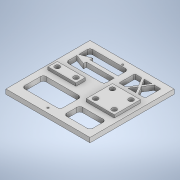
# Autodesk Inventor part: HallSensor_Halterung
Saved by Autodesk Inventor 2022.2 (Build 262287010, 287A)
## iProperties
Created: 2024-01-10
Part Number: HallSensor_Halterung
Material: Generisch
Document SubType Name: Modeling
Designer: ppovolni
Density: 1 g/cm^3
Appearance: Vorgabe
Author: ppovolni
Autodesk Inventor part; units mm, degrees
ref_plane "YZ Plane" through (0, 0, 0) normal (1, 0, 0) x (0, 1, 0)
ref_plane "Arbeitsebene1" through (-21.4485, 99.4, 5.4) normal (-1, 0, 0) x (0, -0.6026, -0.798)
sketch "center1" plane through (-21.4485, 99.4, 5.4) normal (-1, 0, 0) x (0, -0.6026, -0.798)
  line L0 (125.8462, -4.4299) -> (-42.8597, 122.9603)
  line L1 (111.6965, 152.237) -> (-23.2865, -26.5243)
  point P0 (64.2081, 76.0713)
  constraints: 4 end point, 6 other
ref_plane "Arbeitsebene2" through (53.5515, 27.1, 8) normal (0, 0, -1) x (0, 1, 0)
sketch "center2" plane through (53.5515, 27.1, 8) normal (0, 0, -1) x (0, 1, 0)
  line L0 (0, 239.86) -> (0, -220.81)
  point P0 (-27.1, -53.5515)
  constraints: 2 end point, 1 vertical, 2 other
sketch "Hallsensor" plane through (0, 0, 0) normal (0, 1, 0) x (-1, 0, 0)
  line L0 (21.4485, 13) -> (41.4485, 13) construction
  line L1 (41.4485, 13) -> (41.4485, 3) construction
  line L2 (41.4485, 3) -> (21.4485, 3) construction
  line L3 (21.4485, 3) -> (21.4485, 13) construction
  line L4 (21.4485, -97.7) -> (21.4485, 113.7) construction
  line L5 (-293.4115, 8) -> (167.2585, 8) construction
  line L6 (40.4485, 4) -> (42.4485, 4)
  line L7 (42.4485, 4) -> (42.4485, 2)
  line L8 (42.4485, 2) -> (40.4485, 2)
  line L9 (40.4485, 2) -> (40.4485, 4)
  line L10 (40.4485, 4) -> (42.4485, 2) construction
  line L11 (42.4485, 4) -> (40.4485, 2) construction
  line L12 (22.4485, 4) -> (20.4485, 4)
  line L13 (20.4485, 4) -> (20.4485, 2)
  line L14 (20.4485, 2) -> (22.4485, 2)
  line L15 (22.4485, 2) -> (22.4485, 4)
  line L16 (22.4485, 4) -> (20.4485, 2) construction
  line L17 (20.4485, 4) -> (22.4485, 2) construction
  line L18 (22.4485, 14) -> (20.4485, 14)
  line L19 (20.4485, 14) -> (20.4485, 12)
  line L20 (20.4485, 12) -> (22.4485, 12)
  line L21 (22.4485, 12) -> (22.4485, 14)
  line L22 (22.4485, 14) -> (20.4485, 12) construction
  line L23 (20.4485, 14) -> (22.4485, 12) construction
  line L24 (42.4485, 14) -> (40.4485, 14)
  line L25 (40.4485, 14) -> (40.4485, 12)
  line L26 (40.4485, 12) -> (42.4485, 12)
  line L27 (42.4485, 12) -> (42.4485, 14)
  line L28 (42.4485, 14) -> (40.4485, 12) construction
  line L29 (40.4485, 14) -> (42.4485, 12) construction
  line L30 (51.4485, -1) -> (1.4485, -1) construction
  line L31 (1.4485, -1) -> (1.4485, 17) construction
  line L32 (1.4485, 17) -> (51.4485, 17) construction
  line L33 (51.4485, 17) -> (51.4485, -1) construction
  circle A0 centre (51.4485, 8) radius 1.5
  circle A1 centre (1.4485, -1) radius 1.5
  circle A2 centre (1.4485, 17) radius 1.5
  point P0 (0, 0)
  point P1 (21.4485, 3)
  point P2 (21.4485, 3)
  dimension "d70" = 20
  dimension "d71" = 10
  dimension "d72" = 2
  dimension "d73" = 4
  dimension "d74" = 4
  dimension "d75" = 20
  dimension "d76" = 10
  dimension "d77" = 3
  dimension "d78" = 5
  constraints: 64 end point, 12 midpoint, 12 parallel, 6 equal length, 6 horizontal, 6 perpendicular, 3 centre point, 3 coincident, 2 equal radius, 1 collinear, 1 point on line
  measures "d70" distance of L1.end L2.end
  measures "d71" distance of L0.end L1.end
  measures "d72" distance of L7.end L8.end
  measures "d73" distance from line of point (21.448, 3) L30
  measures "d74" distance from line of L32 point (21.448, 13)
  measures "d75" distance from line of point (21.448, 3) L31
  measures "d76" distance between parallel lines of L33 L1
  measures "d77" diameter of A0
  measures "d78" distance between parallel lines of L5 L2
sketch "Groundplane" plane through (0, 0, 0) normal (0, 1, 0) x (-1, 0, 0)
  line L0 (-293.4115, 8) -> (167.2585, 8) construction
  line L1 (21.4485, -97.7) -> (21.4485, 113.7) construction
  arc A0 (22.4485, -32) -> (20.4485, -32) centre (21.4485, -32) ccw construction
  line L2 (22.4485, -32) -> (20.4485, -32) construction
  line L3 (20.4485, -32) -> (20.4485, -37) construction
  line L4 (20.4485, -37) -> (22.4485, -37) construction
  line L5 (22.4485, -37) -> (22.4485, -32) construction
  arc A1 (20.4485, 48) -> (22.4485, 48) centre (21.4485, 48) ccw construction
  line L6 (20.4485, 48) -> (22.4485, 48) construction
  line L7 (22.4485, 48) -> (22.4485, 53) construction
  line L8 (22.4485, 53) -> (20.4485, 53) construction
  line L9 (20.4485, 53) -> (20.4485, 48) construction
  line L10 (61.4485, -37) -> (-28.5515, -37) construction
  line L11 (-28.5515, -37) -> (-28.5515, 53) construction
  line L12 (-28.5515, 53) -> (61.4485, 53) construction
  line L13 (61.4485, 53) -> (61.4485, -37) construction
  dimension "d87" = 5
  dimension "d88" = 2
  dimension "d89" = 2
  dimension "d90" = 5
  dimension "d91" = 90
  dimension "d92" = 45
  dimension "d97" = 50
  dimension "d98" = 90
  constraints: 24 end point, 6 parallel, 5 point on circle, 4 point on line, 3 horizontal, 3 perpendicular, 2 centre point, 2 collinear, 2 midpoint
  measures "d87" distance of L4.end L2.start
  measures "d88" distance of L3.end L4.end
  measures "d89" distance of L7.end L8.end
  measures "d90" distance of L6.end L7.end
  measures "d91" distance of L12.end L10.start
  measures "d92" distance between parallel lines of L0 L10
  measures "d97" distance between parallel lines of L1 L11
  measures "d98" distance of L10.start L10.end
sketch "Montagepunkte" plane through (0, 0, 0) normal (0, 1, 0) x (-1, 0, 0)
  circle A0 centre (51.4485, 8) radius 1.5 construction
  circle A1 centre (1.4485, -1) radius 1.5 construction
  circle A2 centre (1.4485, 17) radius 1.5 construction
  line L0 (1.4485, -1) -> (-18.5515, -1) construction
  line L1 (-18.5515, -1) -> (-18.5515, 17) construction
  line L2 (-18.5515, 17) -> (1.4485, 17) construction
  line L3 (1.4485, 17) -> (1.4485, -1) construction
  line L4 (51.4485, 8) -> (31.4485, 8) construction
  circle A3 centre (31.4485, 8) radius 1.6
  circle A4 centre (51.4485, 8) radius 1.6
  circle A5 centre (1.4485, -1) radius 1.6
  circle A6 centre (1.4485, 17) radius 1.6
  circle A7 centre (-18.5515, 17) radius 1.6
  circle A8 centre (-18.5515, -1) radius 1.6
  arc A9 (22.4485, -32) -> (20.4485, -32) centre (21.4485, -32) ccw construction
  arc A10 (20.4485, 48) -> (22.4485, 48) centre (21.4485, 48) ccw construction
  circle A11 centre (21.4485, -32) radius 1
  circle A12 centre (21.4485, 48) radius 1
  dimension "d93" = 20
  dimension "d94" = 20
  dimension "d95" = 3.2
  dimension "d96" = 2
  constraints: 10 end point, 8 centre point, 8 coincident, 6 equal radius, 2 horizontal, 2 parallel, 1 perpendicular, 1 point on line
  measures "d93" distance of L0.start L0.end
  measures "d94" distance of L4.start L4.end
  measures "d95" diameter of A4
  measures "d96" diameter of A11
sketch "Skizze5" plane through (0, 0, 0) normal (0, 1, 0) x (-1, 0, 0)
  line L0 (-293.4115, 8) -> (167.2585, 8) construction
  circle A0 centre (21.4485, -32) radius 1 projected
  circle A1 centre (21.4485, 48) radius 1 projected
  line L1 (61.4485, -37) -> (-28.5515, -37) projected
  line L2 (61.4485, 53) -> (61.4485, -37) projected
  line L3 (-28.5515, -37) -> (-28.5515, 53) projected
  line L4 (-28.5515, 53) -> (61.4485, 53) projected
extrude "Extrusion2" add sketch "Skizze5" along normal blind 5
sketch "Skizze6" plane through (0, 5, 0) normal (0, 1, 0) x (1, 0, 0)
  line L0 (-56.4485, -3) -> (-26.4485, -3)
  line L1 (-26.4485, -3) -> (-26.4485, -13)
  line L2 (-26.4485, -13) -> (-56.4485, -13)
  line L3 (-56.4485, -13) -> (-56.4485, -3)
  line L4 (-6.4485, 6) -> (23.5515, 6)
  line L5 (23.5515, 6) -> (23.5515, -22)
  line L6 (23.5515, -22) -> (-6.4485, -22)
  line L7 (-6.4485, -22) -> (-6.4485, 6)
  circle A0 centre (-51.4485, -8) radius 1.6 projected
  circle A1 centre (-31.4485, -8) radius 1.6 projected
  circle A2 centre (-1.4485, -17) radius 1.6 projected
  circle A3 centre (18.5515, -17) radius 1.6 projected
  circle A4 centre (18.5515, 1) radius 1.6 projected
  circle A5 centre (-1.4485, 1) radius 1.6 projected
  point P0 (0, 0)
  dimension "d99" = 5
  dimension "d100" = 5
  dimension "d101" = 5
  dimension "d102" = 5
  dimension "d103" = 5
  dimension "d104" = 5
  dimension "d105" = 5
  dimension "d106" = 5
  constraints: 16 end point, 4 parallel, 2 horizontal, 2 perpendicular
  measures "d99" distance from line of A0.centre L0
  measures "d100" distance from line of L2 A0.centre
  measures "d101" distance from line of A1.centre L1
  measures "d102" distance from line of L3 A0.centre
  measures "d103" distance from line of L7 A5.centre
  measures "d104" distance from line of L5 A4.centre
  measures "d105" distance from line of A4.centre L4
  measures "d106" distance from line of L6 A3.centre
extrude "Extrusion3" add sketch "Skizze6" along normal blind 3
chamfer "Fase1" distance 1 distance2 3 2 edges at (-53.0485, 8, 8) (-33.0485, 8, 8) measured on face at (-38.3043, 8, 4.168)
chamfer "Fase2" distance 1 distance2 3 4 edges at (-3.0485, 8, -1) (16.9515, 8, -1) (16.9515, 8, 17) (-3.0485, 8, 17) measured on face at (11.4857, 8, 5.3537)
sketch "Skizze7" plane through (0, 5, 0) normal (0, 1, 0) x (1, 0, 0)
  line L0 (-51.4505, 30) -> (-16.4485, 30)
  line L1 (-13.4485, 27) -> (-13.4485, 7)
  line L2 (-16.4485, 4) -> (-51.4505, 4)
  line L3 (-54.4505, 7) -> (-54.4505, 27)
  line L4 (-51.4505, -20) -> (-16.4485, -20)
  line L5 (-13.4485, -23) -> (-13.4485, -40)
  line L6 (-16.4485, -43) -> (-51.4505, -43)
  line L7 (-54.4505, -40) -> (-54.4505, -23)
  line L8 (-3.4485, -29) -> (18.5497, -29)
  line L9 (21.5497, -32) -> (21.5497, -43)
  line L10 (18.5497, -46) -> (-3.4485, -46)
  line L11 (-6.4485, -43) -> (-6.4485, -32)
  line L12 (28.5497, -53) -> (28.5497, 37)
  line L13 (-61.4505, -53) -> (28.5497, -53)
  line L14 (-61.4505, 37) -> (-61.4505, -53)
  line L15 (-56.4485, -13) -> (-26.4485, -13) projected
  line L16 (-6.4485, 6) -> (-6.4485, -22) projected
  line L17 (-26.4485, -3) -> (-56.4485, -3) projected
  line L18 (28.5497, 37) -> (-61.4505, 37)
  line L19 (-6.4485, -22) -> (23.5515, -22) projected
  line L20 (-5.4485, 30) -> (20.5497, 30)
  line L21 (21.5497, 29) -> (21.5497, 14)
  line L22 (20.5497, 13) -> (-5.4485, 13)
  line L23 (-6.4485, 14) -> (-6.4485, 29)
  line L24 (23.5515, 6) -> (-6.4485, 6) projected
  arc A0 (-51.4505, 30) -> (-54.4505, 27) centre (-51.4505, 27) ccw
  arc A1 (-54.4505, 7) -> (-51.4505, 4) centre (-51.4505, 7) ccw
  arc A2 (-13.4485, 27) -> (-16.4485, 30) centre (-16.4485, 27) ccw
  arc A3 (-16.4485, 4) -> (-13.4485, 7) centre (-16.4485, 7) ccw
  arc A4 (-51.4505, -20) -> (-54.4505, -23) centre (-51.4505, -23) ccw
  arc A5 (-13.4485, -23) -> (-16.4485, -20) centre (-16.4485, -23) ccw
  arc A6 (-16.4485, -43) -> (-13.4485, -40) centre (-16.4485, -40) ccw
  arc A7 (-54.4505, -40) -> (-51.4505, -43) centre (-51.4505, -40) ccw
  arc A8 (-3.4485, -29) -> (-6.4485, -32) centre (-3.4485, -32) ccw
  arc A9 (-6.4485, -43) -> (-3.4485, -46) centre (-3.4485, -43) ccw
  arc A10 (18.5497, -46) -> (21.5497, -43) centre (18.5497, -43) ccw
  arc A11 (21.5497, -32) -> (18.5497, -29) centre (18.5497, -32) ccw
  arc A12 (-5.4485, 30) -> (-6.4485, 29) centre (-5.4485, 29) ccw
  arc A13 (-6.4485, 14) -> (-5.4485, 13) centre (-5.4485, 14) ccw
  arc A14 (21.5497, 29) -> (20.5497, 30) centre (20.5497, 29) ccw
  arc A15 (20.5497, 13) -> (21.5497, 14) centre (20.5497, 14) ccw
  point P0 (0, 0)
  point P1 (-13.4485, -43)
  point P2 (-41.4485, -3)
  point P3 (-6.4485, -37.5)
  point P4 (-6.4485, 21.5)
  dimension "d42" = 7
  dimension "d43" = 7
  dimension "d44" = 7
  dimension "d45" = 10
  dimension "d46" = 7
  dimension "d47" = 7
  dimension "d48" = 7
  dimension "d49" = 7
  dimension "d50" = 7
  dimension "d51" = 7
  dimension "d52" = 7
  dimension "d53" = 7
  dimension "d54" = 7
  dimension "d55" = 7
  dimension "d56" = 7
  dimension "d57" = 7
  dimension "d58" = 3
  dimension "d59" = 3
  dimension "d60" = 1
  constraints: 40 end point, 32 point on circle, 32 tangent, 16 centre point, 13 equal radius, 8 parallel, 4 horizontal, 4 perpendicular, 3 midpoint, 3 point on line
  measures "d42" distance between parallel lines of L9 L12
  measures "d43" distance between parallel lines of L13 L10
  measures "d44" distance between parallel lines of L14 L7
  measures "d45" distance between parallel lines of L13 L6
  measures "d46" distance between parallel lines of L4 L15
  measures "d47" distance between parallel lines of L5 L16
  measures "d48" distance from line of point (-41.448, -3) L2
  measures "d49" distance between parallel lines of L14 L3
  measures "d50" distance between parallel lines of L0 L18
  measures "d51" distance between parallel lines of L1 L16
  measures "d52" distance between parallel lines of L8 L19
  measures "d53" distance from line of point (-6.448, -37.5) L5
  measures "d54" distance between parallel lines of L20 L18
  measures "d55" distance between parallel lines of L12 L21
  measures "d56" distance between parallel lines of L24 L22
  measures "d57" distance from line of point (-6.448, 21.5) L1
  measures "d58" radius of A0
  measures "d59" radius of A4
  measures "d60" radius of A12
extrude "Extrusion4" cut sketch "Skizze7" against normal through all contours L0 A2 L1 A3 L2 A1 L3 A0 | L4 A5 L5 A6 L6 A7 L7 A4 | L8 A11 L9 A10 L10 A9 L11 A8 | L20 A14 L21 A15 L22 A13 L23 A12
sketch "Skizze11" plane through (0, 5, 0) normal (0, 1, 0) x (1, 0, 0)
  line L0 (-54.4505, 7) -> (-54.4505, 27) projected
  line L1 (-13.4485, 27) -> (-13.4485, 7) projected
  line L2 (20.5497, 13) -> (-5.4485, 13) construction
  line L3 (-54.4505, 18) -> (-43.4485, 22)
  line L4 (-43.4485, 22) -> (-43.4485, 19)
  line L5 (-43.4485, 19) -> (-13.4485, 19)
  line L6 (-54.4505, 16) -> (-43.4485, 12)
  line L7 (-43.4485, 12) -> (-43.4485, 15)
  line L8 (-43.4485, 15) -> (-13.4485, 15)
  line L9 (14.239, 13) -> (11.6491, 13)
  line L10 (11.6491, 13) -> (7.5162, 19.778)
  line L11 (7.5162, 19.778) -> (3.3006, 13)
  line L12 (3.3006, 13) -> (0.8622, 13)
  line L13 (0.8622, 13) -> (6.2763, 21.5138)
  line L14 (6.2763, 21.5138) -> (1.0275, 30)
  line L15 (1.0275, 30) -> (3.6175, 30)
  line L16 (3.6175, 30) -> (7.6677, 23.346)
  line L17 (7.6677, 23.346) -> (11.8006, 30)
  line L18 (11.8006, 30) -> (14.239, 30)
  line L19 (14.239, 30) -> (8.9214, 21.624)
  line L20 (8.9214, 21.624) -> (14.239, 13)
  point P0 (0, 0)
  point P1 (-54.4505, 17)
  point P2 (-54.4505, 17)
  point P3 (-54.4505, 17)
  point P4 (-54.4505, 17)
  point P5 (-54.4505, 17)
  dimension "d108" = 4
  dimension "d109" = 2
  dimension "d110" = 30
  dimension "d111" = 3
  dimension "d112" = 3
  dimension "d113" = 1
  dimension "d114" = 1
  constraints: 12 end point, 4 point on line, 2 perpendicular, 1 horizontal, 1 vertical, 8 other
  measures "d108" distance between parallel lines of L8 L5
  measures "d109" distance from line of point (-54.45, 17) L5
  measures "d110" distance of L4.end L5.end
  measures "d111" distance of L3.end L4.end
  measures "d112" distance of L6.end L7.end
  measures "d113" distance of point (-54.45, 17) L3.start
  measures "d114" distance of L6.start point (-54.45, 17)
extrude "Extrusion5" add sketch "Skizze11" against normal up to surface (5 mm away)
